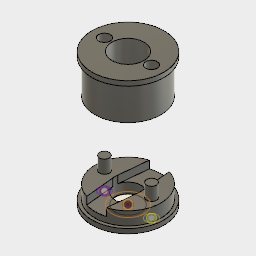
Drive Wheel (Autodesk Fusion 360 design; units mm, degrees)
Autodesk Fusion 360 part; units mm, degrees
sketch "Hub (top)" plane through (0, 0, 0) normal (0, 1, 0) x (1, 0, 0)
  circle A0 centre (0, 0) radius 8.89
  dimension "d1" = 17.78
  measures "d1" diameter of A0
extrude "Extrude1" add sketch "Hub (top)" along normal blind 10.414 makes body 1
sketch "End Cap (top" plane through (0, 10.414, 0) normal (0, 1, 0) x (-1, 0, 0)
  circle A0 centre (0, 0) radius 8.89
  circle A1 centre (0, 0) radius 9.7155
  dimension "d4" = 19.431
  measures "d4" diameter of A1
extrude "Extrude2" add sketch "End Cap (top" against normal blind 1.27 contours A0 | A1 bodies 1
sketch "Bore (top)" plane through (0, 0, 0) normal (0, 1, 0) x (-1, 0, 0)
  circle A0 centre (0, 0) radius 4.318
  line L0 (13.97, 0) -> (-15.662, 0) construction
  circle A1 centre (-6.35, 0) radius 1.5494
  circle A2 centre (6.35, 0) radius 1.5494
  dimension "d16" = 8.636
  dimension "d17" = 3.0988
  dimension "d18" = 3.0988
  dimension "d19" = 6.35
  dimension "d20" = 6.35
  measures "d16" diameter of A0
  measures "d17" diameter of A2
  measures "d18" diameter of A1
  measures "d19" distance of A0.centre A2.centre
  measures "d20" distance of A0.centre A1.centre
extrude "Extrude3" cut sketch "Bore (top)" along normal blind 15.24 bodies 1
ref_plane "WorkPlane1" through (0, -25.4, 0) normal (0, -1, 0) x (-1, 0, 0) in component "Component"
sketch "Hub (bottom)" plane through (0, -25.4, 0) normal (0, -1, 0) x (1, 0, 0) in component "Component"
  circle A0 centre (0, 0) radius 8.89
  circle A1 centre (0, 0) radius 8.89
  dimension "d24" = 17.78
  measures "d24" diameter of A0
extrude "Extrude1'" add sketch "Hub (bottom)" against normal blind 4.826 separate body makes body 2 in component "Component"
sketch "End Cap (bottoom)" plane through (0, -25.4, 0) normal (0, -1, 0) x (1, 0, 0) in component "Component"
  circle A0 centre (0, 0) radius 9.7155
  circle A1 centre (0, 0) radius 9.7155
  dimension "d27" = 19.431
  measures "d27" diameter of A0
extrude "Extrude2'" add sketch "End Cap (bottoom)" against normal blind 1.27 bodies 2 in component "Component"
sketch "Posts" plane through (0, -25.4, 0) normal (0, -1, 0) x (1, 0, 0) in component "Component"
  circle A0 centre (0, 0) radius 3.4925
  circle A1 centre (0, 0) radius 4.318
  circle A2 centre (0, 0) radius 4.318
  circle A3 centre (6.35, 0) radius 1.3335
  circle A4 centre (6.35, 0) radius 1.5494
  circle A5 centre (-6.35, 0) radius 1.3335
  circle A6 centre (-6.35, 0) radius 1.5494
  dimension "d46" = 2.667
  dimension "d47" = 2.667
  dimension "d48" = 6.985
  measures "d46" diameter of A5
  measures "d47" diameter of A3
  measures "d48" diameter of A0
extrude "Extrude7" cut sketch "Posts" against normal blind 5.842 contours A0 bodies 2 in component "Component"
extrude "Extrude4" add sketch "Posts" against normal blind 8.382 contours A3 | A5 bodies 2 in component "Component"
sketch "Sketch4" plane through (0, -20.574, 0) normal (0, 1, 0) x (-1, 0, 0)
  circle A0 centre (-6.35, 0) radius 1.3335
  circle A1 centre (6.35, 0) radius 1.3335
  circle A2 centre (0, 0) radius 3.4925
  circle A3 centre (0, 0) radius 8.89
  line L0 (0, -15.24) -> (0, 14.5261) construction
  line L1 (-2.667, 11.581) -> (2.667, 11.581) construction
  line L2 (2.667, 11.581) -> (2.667, -11.581) construction
  line L3 (2.667, -11.581) -> (-2.667, -11.581) construction
  line L4 (-2.667, -11.581) -> (-2.667, 11.581) construction
  line L5 (-2.667, 11.581) -> (2.667, -11.581) construction
  line L6 (2.667, 11.581) -> (-2.667, -11.581) construction
  line L7 (3.4925, 0) -> (2.667, -8.4805)
  line L8 (2.667, -8.4805) -> (2.4196, -11.0222)
  line L9 (-3.4925, 0.0073) -> (-2.667, -8.4805)
  line L10 (-2.667, -8.4805) -> (-2.0817, -11.0222)
  line L11 (-2.0817, -11.0222) -> (2.4196, -11.0222)
  line L12 (3.4925, 0) -> (2.667, 8.4805)
  line L13 (-3.4925, 0.0073) -> (-2.667, 8.4805)
  line L14 (-2.667, 8.4805) -> (-2.4547, 10.6593)
  line L15 (2.4547, 10.6593) -> (2.667, 8.4805)
  line L16 (2.4547, 10.6593) -> (-2.4547, 10.6593)
  point P0 (3.4925, 0)
  dimension "d51" = 5.334
  measures "d51" distance of L2.end L3.end
extrude "Extrude8" cut sketch "Sketch4" against normal blind 2.032 contours A2 A3 L12 L13 | A2 A3 L7 L9 bodies 2 in component "Component"
component "Component" placed x (1, 0, 0) y (0, 1, 0) z (0, 0, 1) at (0, 0, 0)
equation "d2 = 0.6 in - 0.11 in - 0.08 in"
equation "capEnd = 0.765 in"
equation "bore = 0.340 in"
equation "post = 0.105 in"
equation "postHole = 0.122 in"
equation "postdist = 0.25 in"
equation "servoArmHole = 0.225 in"
equation "armDepth = 0.8 in"
equation "capThickness = 0.05 in"
equation "d16 = bore"
equation "d17 = postHole"
equation "d18 = postHole"
equation "d19 = postdist"
equation "d20 = postdist"
equation "d25 = -0.11 in - 0.08 in"
equation "d46 = post"
equation "d47 = post"
equation "d52 = -0.19 in + 0.11 in"
